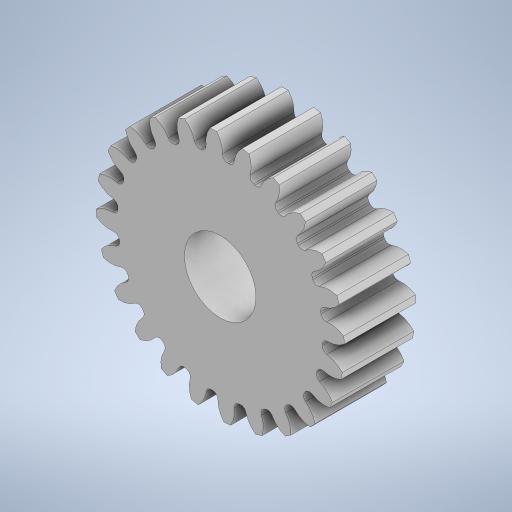
# Autodesk Inventor part: Spur_Gear_24
Saved by Autodesk Inventor 2024 (Build 280153000, 153)
## iProperties
Created: 2024-10-23
Part Number: Spur_Gear_24
Material: Generic
Document SubType Name: Modeling
Designer: Yash Purswani
Density: 1 g/cm^3
Appearance: Default
Author: Yash Purswani
Autodesk Inventor part; units mm, degrees
ref_plane "YZ Plane" through (0, 0, 0) normal (1, 0, 0) x (0, 1, 0)
ref_plane "XZ Plane" through (0, 0, 0) normal (0, 1, 0) x (-1, 0, 0)
ref_plane "XY Plane" through (0, 0, 0) normal (0, 0, 1) x (1, 0, 0)
sketch "Sketch1" plane through (0, 0, 0) normal (0, 0, 1) x (1, 0, 0)
  arc A0 (0.4815, 22.5475) -> (-0.7187, 25.9901) centre (-4.7363, 22.6589) ccw
  arc A1 (-2.1666, 25.9096) -> (-2.9778, 22.3552) centre (2.1955, 23.0443) ccw
  arc A2 (-3.8301, 21.1561) -> (-2.9778, 22.3552) centre (-4.0177, 22.1919) ccw
  arc A3 (0.4815, 22.5475) -> (1.4615, 21.4503) centre (1.5331, 22.5005) ccw
  arc A4 (-8.7987, 24.466) -> (-8.6623, 20.8227) centre (-3.8436, 22.8273) ccw
  arc A5 (-5.3706, 21.9038) -> (-7.4209, 24.9185) centre (-10.4395, 20.661) ccw
  arc A6 (-5.3706, 21.9038) -> (-4.14, 21.0976) centre (-4.3427, 22.1306) ccw
  arc A7 (-9.1752, 19.4439) -> (-8.6623, 20.8227) centre (-9.6245, 20.3959) ccw
  arc A8 (-14.8311, 21.355) -> (-13.7564, 17.8712) centre (-9.6208, 21.0547) ccw
  arc A9 (-10.8568, 19.7674) -> (-13.6174, 22.1487) centre (-15.4312, 17.255) ccw
  arc A10 (-10.8568, 19.7674) -> (-9.4594, 19.3072) centre (-9.9226, 20.2525) ccw
  arc A11 (-13.895, 16.4066) -> (-13.7564, 17.8712) centre (-14.5753, 17.2099) ccw
  arc A12 (-19.8528, 16.7888) -> (-17.9131, 13.7019) centre (-14.7423, 17.8472) ccw
  arc A13 (-15.603, 16.2839) -> (-18.8859, 17.8696) centre (-19.3713, 12.6732) ccw
  arc A14 (-15.603, 16.2839) -> (-14.1342, 16.2011) centre (-14.8262, 16.9943) ccw
  arc A15 (-17.6679, 12.2513) -> (-17.9131, 13.7019) centre (-18.5329, 12.8511) ccw
  arc A16 (-23.5216, 11.0785) -> (-20.849, 8.5987) centre (-18.8592, 13.4235) ccw
  arc A17 (-19.2859, 11.6907) -> (-22.8674, 12.3726) centre (-21.9913, 7.2277) ccw
  arc A18 (-19.2859, 11.6907) -> (-17.8457, 11.9908) centre (-18.7194, 12.5779) ccw
  arc A19 (-20.2368, 7.261) -> (-20.849, 8.5987) centre (-21.2276, 7.6165) ccw
  arc A20 (-25.5875, 4.6131) -> (-22.3641, 2.9096) centre (-21.6908, 8.085) ccw
  arc A21 (-21.6546, 6.3008) -> (-25.2905, 6.0325) centre (-23.1127, 1.2896) ccw
  arc A22 (-21.6546, 6.3008) -> (-20.3411, 6.9635) centre (-21.337, 7.3044) ccw
  arc A23 (-21.4265, 1.776) -> (-22.3641, 2.9096) centre (-22.4756, 1.8629) ccw
  arc A24 (-25.9096, -2.1666) -> (-22.3552, -2.9778) centre (-23.0443, 2.1955) ccw
  arc A25 (-22.5475, 0.4815) -> (-25.9901, -0.7187) centre (-22.6589, -4.7363) ccw
  arc A26 (-22.5475, 0.4815) -> (-21.4503, 1.4615) centre (-22.5005, 1.5331) ccw
  arc A27 (-21.1561, -3.8301) -> (-22.3552, -2.9778) centre (-22.1919, -4.0177) ccw
  arc A28 (-24.466, -8.7987) -> (-20.8227, -8.6623) centre (-22.8273, -3.8436) ccw
  arc A29 (-21.9038, -5.3706) -> (-24.9185, -7.4209) centre (-20.661, -10.4395) ccw
  arc A30 (-21.9038, -5.3706) -> (-21.0976, -4.14) centre (-22.1306, -4.3427) ccw
  arc A31 (-19.4439, -9.1752) -> (-20.8227, -8.6623) centre (-20.3959, -9.6245) ccw
  arc A32 (-21.355, -14.8311) -> (-17.8712, -13.7564) centre (-21.0547, -9.6208) ccw
  arc A33 (-19.7674, -10.8568) -> (-22.1487, -13.6174) centre (-17.255, -15.4312) ccw
  arc A34 (-19.7674, -10.8568) -> (-19.3072, -9.4594) centre (-20.2525, -9.9226) ccw
  arc A35 (-16.4066, -13.895) -> (-17.8712, -13.7564) centre (-17.2099, -14.5753) ccw
  arc A36 (-16.7888, -19.8528) -> (-13.7019, -17.9131) centre (-17.8472, -14.7423) ccw
  arc A37 (-16.2839, -15.603) -> (-17.8696, -18.8859) centre (-12.6732, -19.3713) ccw
  arc A38 (-16.2839, -15.603) -> (-16.2011, -14.1342) centre (-16.9943, -14.8262) ccw
  arc A39 (-12.2513, -17.6679) -> (-13.7019, -17.9131) centre (-12.8511, -18.5329) ccw
  arc A40 (-11.0785, -23.5216) -> (-8.5987, -20.849) centre (-13.4235, -18.8592) ccw
  arc A41 (-11.6907, -19.2859) -> (-12.3726, -22.8674) centre (-7.2277, -21.9913) ccw
  arc A42 (-11.6907, -19.2859) -> (-11.9908, -17.8457) centre (-12.5779, -18.7194) ccw
  arc A43 (-7.261, -20.2368) -> (-8.5987, -20.849) centre (-7.6165, -21.2276) ccw
  arc A44 (-4.6131, -25.5875) -> (-2.9096, -22.3641) centre (-8.085, -21.6908) ccw
  arc A45 (-6.3008, -21.6546) -> (-6.0325, -25.2905) centre (-1.2896, -23.1127) ccw
  arc A46 (-6.3008, -21.6546) -> (-6.9635, -20.3411) centre (-7.3044, -21.337) ccw
  arc A47 (-1.776, -21.4265) -> (-2.9096, -22.3641) centre (-1.8629, -22.4756) ccw
  arc A48 (2.1666, -25.9096) -> (2.9778, -22.3552) centre (-2.1955, -23.0443) ccw
  arc A49 (-0.4815, -22.5475) -> (0.7187, -25.9901) centre (4.7363, -22.6589) ccw
  arc A50 (-0.4815, -22.5475) -> (-1.4615, -21.4503) centre (-1.5331, -22.5005) ccw
  arc A51 (3.8301, -21.1561) -> (2.9778, -22.3552) centre (4.0177, -22.1919) ccw
  arc A52 (8.7987, -24.466) -> (8.6623, -20.8227) centre (3.8436, -22.8273) ccw
  arc A53 (5.3706, -21.9038) -> (7.4209, -24.9185) centre (10.4395, -20.661) ccw
  arc A54 (5.3706, -21.9038) -> (4.14, -21.0976) centre (4.3427, -22.1306) ccw
  arc A55 (9.1752, -19.4439) -> (8.6623, -20.8227) centre (9.6245, -20.3959) ccw
  arc A56 (14.8311, -21.355) -> (13.7564, -17.8712) centre (9.6208, -21.0547) ccw
  arc A57 (10.8568, -19.7674) -> (13.6174, -22.1487) centre (15.4312, -17.255) ccw
  arc A58 (10.8568, -19.7674) -> (9.4594, -19.3072) centre (9.9226, -20.2525) ccw
  arc A59 (13.895, -16.4066) -> (13.7564, -17.8712) centre (14.5753, -17.2099) ccw
  arc A60 (19.8528, -16.7888) -> (17.9131, -13.7019) centre (14.7423, -17.8472) ccw
  arc A61 (15.603, -16.2839) -> (18.8859, -17.8696) centre (19.3713, -12.6732) ccw
  arc A62 (15.603, -16.2839) -> (14.1342, -16.2011) centre (14.8262, -16.9943) ccw
  arc A63 (17.6679, -12.2513) -> (17.9131, -13.7019) centre (18.5329, -12.8511) ccw
  arc A64 (23.5216, -11.0785) -> (20.849, -8.5987) centre (18.8592, -13.4235) ccw
  arc A65 (19.2859, -11.6907) -> (22.8674, -12.3726) centre (21.9913, -7.2277) ccw
  arc A66 (19.2859, -11.6907) -> (17.8457, -11.9908) centre (18.7194, -12.5779) ccw
  arc A67 (20.2368, -7.261) -> (20.849, -8.5987) centre (21.2276, -7.6165) ccw
  arc A68 (25.5875, -4.6131) -> (22.3641, -2.9096) centre (21.6908, -8.085) ccw
  arc A69 (21.6546, -6.3008) -> (25.2905, -6.0325) centre (23.1127, -1.2896) ccw
  arc A70 (21.6546, -6.3008) -> (20.3411, -6.9635) centre (21.337, -7.3044) ccw
  arc A71 (21.4265, -1.776) -> (22.3641, -2.9096) centre (22.4756, -1.8629) ccw
  arc A72 (25.9096, 2.1666) -> (22.3552, 2.9778) centre (23.0443, -2.1955) ccw
  arc A73 (22.5475, -0.4815) -> (25.9901, 0.7187) centre (22.6589, 4.7363) ccw
  arc A74 (22.5475, -0.4815) -> (21.4503, -1.4615) centre (22.5005, -1.5331) ccw
  arc A75 (21.1561, 3.8301) -> (22.3552, 2.9778) centre (22.1919, 4.0177) ccw
  arc A76 (24.466, 8.7987) -> (20.8227, 8.6623) centre (22.8273, 3.8436) ccw
  arc A77 (21.9038, 5.3706) -> (24.9185, 7.4209) centre (20.661, 10.4395) ccw
  arc A78 (21.9038, 5.3706) -> (21.0976, 4.14) centre (22.1306, 4.3427) ccw
  arc A79 (19.4439, 9.1752) -> (20.8227, 8.6623) centre (20.3959, 9.6245) ccw
  arc A80 (21.355, 14.8311) -> (17.8712, 13.7564) centre (21.0547, 9.6208) ccw
  arc A81 (19.7674, 10.8568) -> (22.1487, 13.6174) centre (17.255, 15.4312) ccw
  arc A82 (19.7674, 10.8568) -> (19.3072, 9.4594) centre (20.2525, 9.9226) ccw
  arc A83 (16.4066, 13.895) -> (17.8712, 13.7564) centre (17.2099, 14.5753) ccw
  arc A84 (16.7888, 19.8528) -> (13.7019, 17.9131) centre (17.8472, 14.7423) ccw
  arc A85 (16.2839, 15.603) -> (17.8696, 18.8859) centre (12.6732, 19.3713) ccw
  arc A86 (16.2839, 15.603) -> (16.2011, 14.1342) centre (16.9943, 14.8262) ccw
  arc A87 (12.2513, 17.6679) -> (13.7019, 17.9131) centre (12.8511, 18.5329) ccw
  arc A88 (11.0785, 23.5216) -> (8.5987, 20.849) centre (13.4235, 18.8592) ccw
  arc A89 (11.6907, 19.2859) -> (12.3726, 22.8674) centre (7.2277, 21.9913) ccw
  arc A90 (11.6907, 19.2859) -> (11.9908, 17.8457) centre (12.5779, 18.7194) ccw
  arc A91 (7.261, 20.2368) -> (8.5987, 20.849) centre (7.6165, 21.2276) ccw
  arc A92 (4.6131, 25.5875) -> (2.9096, 22.3641) centre (8.085, 21.6908) ccw
  arc A93 (6.3008, 21.6546) -> (6.0325, 25.2905) centre (1.2896, 23.1127) ccw
  arc A94 (6.3008, 21.6546) -> (6.9635, 20.3411) centre (7.3044, 21.337) ccw
  arc A95 (1.776, 21.4265) -> (2.9096, 22.3641) centre (1.8629, 22.4756) ccw
  arc A96 (-0.7187, 25.9901) -> (-2.1666, 25.9096) centre (0, 0) ccw
  arc A97 (6.0325, 25.2905) -> (4.6131, 25.5875) centre (0, 0) ccw
  arc A98 (12.3726, 22.8674) -> (11.0785, 23.5216) centre (0, 0) ccw
  arc A99 (17.8696, 18.8859) -> (16.7888, 19.8528) centre (0, 0) ccw
  arc A100 (22.1487, 13.6174) -> (21.355, 14.8311) centre (0, 0) ccw
  arc A101 (24.9185, 7.4209) -> (24.466, 8.7987) centre (0, 0) ccw
  arc A102 (25.9901, 0.7187) -> (25.9096, 2.1666) centre (0, 0) ccw
  arc A103 (25.2905, -6.0325) -> (25.5875, -4.6131) centre (0, 0) ccw
  arc A104 (22.8674, -12.3726) -> (23.5216, -11.0785) centre (0, 0) ccw
  arc A105 (1.776, 21.4265) -> (1.4615, 21.4503) centre (0, 0) ccw
  arc A106 (-3.8301, 21.1561) -> (-4.14, 21.0976) centre (0, 0) ccw
  arc A107 (-9.1752, 19.4439) -> (-9.4594, 19.3072) centre (0, 0) ccw
  arc A108 (-13.895, 16.4066) -> (-14.1342, 16.2011) centre (0, 0) ccw
  arc A109 (-17.6679, 12.2513) -> (-17.8457, 11.9908) centre (0, 0) ccw
  arc A110 (-20.2368, 7.261) -> (-20.3411, 6.9635) centre (0, 0) ccw
  arc A111 (-21.4265, 1.776) -> (-21.4503, 1.4615) centre (0, 0) ccw
  arc A112 (-22.8674, 12.3726) -> (-23.5216, 11.0785) centre (0, 0) ccw
  arc A113 (-18.8859, 17.8696) -> (-19.8528, 16.7888) centre (0, 0) ccw
  arc A114 (-7.4209, 24.9185) -> (-8.7987, 24.466) centre (0, 0) ccw
  arc A115 (-13.6174, 22.1487) -> (-14.8311, 21.355) centre (0, 0) ccw
  arc A116 (-25.2905, 6.0325) -> (-25.5875, 4.6131) centre (0, 0) ccw
  arc A117 (-25.9901, -0.7187) -> (-25.9096, -2.1666) centre (0, 0) ccw
  arc A118 (-24.9185, -7.4209) -> (-24.466, -8.7987) centre (0, 0) ccw
  arc A119 (-22.1487, -13.6174) -> (-21.355, -14.8311) centre (0, 0) ccw
  arc A120 (-17.8696, -18.8859) -> (-16.7888, -19.8528) centre (0, 0) ccw
  arc A121 (-21.1561, -3.8301) -> (-21.0976, -4.14) centre (0, 0) ccw
  arc A122 (-19.4439, -9.1752) -> (-19.3072, -9.4594) centre (0, 0) ccw
  arc A123 (-16.4066, -13.895) -> (-16.2011, -14.1342) centre (0, 0) ccw
  arc A124 (-12.2513, -17.6679) -> (-11.9908, -17.8457) centre (0, 0) ccw
  arc A125 (-7.261, -20.2368) -> (-6.9635, -20.3411) centre (0, 0) ccw
  arc A126 (-1.776, -21.4265) -> (-1.4615, -21.4503) centre (0, 0) ccw
  arc A127 (3.8301, -21.1561) -> (4.14, -21.0976) centre (0, 0) ccw
  arc A128 (9.1752, -19.4439) -> (9.4594, -19.3072) centre (0, 0) ccw
  arc A129 (13.895, -16.4066) -> (14.1342, -16.2011) centre (0, 0) ccw
  arc A130 (17.6679, -12.2513) -> (17.8457, -11.9908) centre (0, 0) ccw
  arc A131 (20.2368, -7.261) -> (20.3411, -6.9635) centre (0, 0) ccw
  arc A132 (21.4265, -1.776) -> (21.4503, -1.4615) centre (0, 0) ccw
  arc A133 (21.1561, 3.8301) -> (21.0976, 4.14) centre (0, 0) ccw
  arc A134 (19.4439, 9.1752) -> (19.3072, 9.4594) centre (0, 0) ccw
  arc A135 (16.4066, 13.895) -> (16.2011, 14.1342) centre (0, 0) ccw
  arc A136 (12.2513, 17.6679) -> (11.9908, 17.8457) centre (0, 0) ccw
  arc A137 (7.261, 20.2368) -> (6.9635, 20.3411) centre (0, 0) ccw
  arc A138 (18.8859, -17.8696) -> (19.8528, -16.7888) centre (0, 0) ccw
  arc A139 (13.6174, -22.1487) -> (14.8311, -21.355) centre (0, 0) ccw
  arc A140 (-12.3726, -22.8674) -> (-11.0785, -23.5216) centre (0, 0) ccw
  arc A141 (-6.0325, -25.2905) -> (-4.6131, -25.5875) centre (0, 0) ccw
  arc A142 (0.7187, -25.9901) -> (2.1666, -25.9096) centre (0, 0) ccw
  arc A143 (7.4209, -24.9185) -> (8.7987, -24.466) centre (0, 0) ccw
  circle A144 centre (0, 0) radius 7.5
  dimension "d15" = 360
  dimension "d17" = 15
  constraints: 288 point on circle, 145 centre point, 2 coincident, 337 other
  measures "d17" diameter of A144
extrude "Extrusion1" add sketch "Sketch1" along normal blind 15
body "Solid1"
